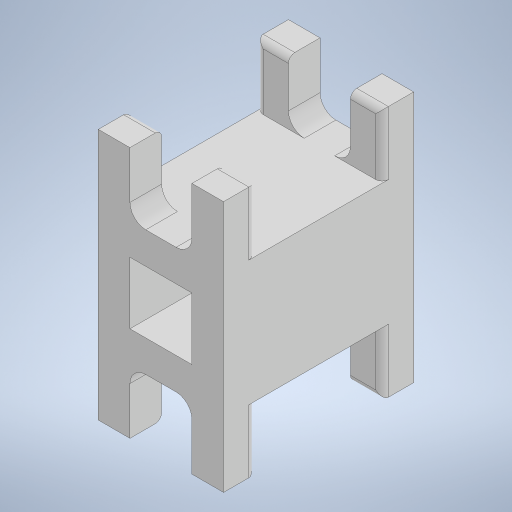
# Autodesk Inventor part: zigu3
Saved by Autodesk Inventor 2024.3 (Build 283343010, 343A)
## iProperties
Created: 2025-10-22
Part Number: zigu3
Material: 一般
Document SubType Name: Modeling
Designer: kshau
Density: 1 g/cm^3
Appearance: 既定
Author: kshau
Autodesk Inventor part; units mm, degrees
ref_plane "YZ Plane" through (0, 0, 0) normal (1, 0, 0) x (0, 1, 0)
ref_plane "XZ Plane" through (0, 0, 0) normal (0, 1, 0) x (-1, 0, 0)
ref_plane "XY Plane" through (0, 0, 0) normal (0, 0, 1) x (1, 0, 0)
sketch "スケッチ1" plane through (0, 0, 0) normal (0, 0, 1) x (1, 0, 0)
  line L0 (0, 0) -> (39.6, 0)
  line L1 (39.6, 0) -> (39.6, 39.6)
  line L2 (39.6, 39.6) -> (0, 39.6)
  line L3 (0, 39.6) -> (0, 0)
  line L4 (10, 29.6) -> (29.6, 29.6)
  line L5 (29.6, 29.6) -> (29.6, 10)
  line L6 (29.6, 10) -> (10, 10)
  line L7 (10, 10) -> (10, 29.6)
  dimension "d0" = 39.6
  dimension "d1" = 39.6
  dimension "d2" = 10
  dimension "d3" = 10
  dimension "d4" = 10
  dimension "d5" = 10
  constraints: 16 end point, 4 parallel, 2 horizontal, 2 perpendicular
  measures "d0" distance of L0.end L1.end
  measures "d1" distance of L1.end L2.end
  measures "d2" distance between parallel lines of L3 L7
  measures "d3" distance between parallel lines of L1 L5
  measures "d4" distance between parallel lines of L0 L6
  measures "d5" distance between parallel lines of L2 L4
extrude "押し出し1" add sketch "スケッチ1" along normal blind 20.05
sketch "スケッチ2" plane through (0, 0, 20.05) normal (0, 0, 1) x (1, 0, 0)
  line L0 (10, 10) -> (10, 29.6) projected
  line L1 (29.6, 29.6) -> (29.6, 10) projected
  line L2 (10, 10) -> (29.6, 10)
  line L3 (29.6, 10) -> (29.6, 29.6)
  line L4 (29.6, 29.6) -> (10, 29.6)
  line L5 (10, 29.6) -> (10, 10)
  line L6 (39.6, 39.6) -> (0, 39.6) projected
  line L7 (0, 39.6) -> (39.6, 39.6)
  line L8 (39.6, 39.6) -> (39.6, -20)
  line L9 (39.6, -20) -> (0, -20)
  line L10 (0, -20) -> (0, 39.6)
  line L11 (0, 0) -> (39.6, 0) projected
  line L12 (10, -20) -> (29.6, -20)
  line L13 (29.6, -20) -> (29.6, 0)
  line L14 (29.6, 0) -> (10, 0)
  line L15 (10, 0) -> (10, -20)
  line L16 (0, 0) -> (39.6, 0)
  line L17 (39.6, 0) -> (39.6, 59.6)
  line L18 (39.6, 59.6) -> (0, 59.6)
  line L19 (0, 59.6) -> (0, 0)
  line L20 (10, -20) -> (29.6, -20)
  line L21 (29.6, -20) -> (29.6, 59.6)
  line L22 (29.6, 59.6) -> (10, 59.6)
  line L23 (10, 59.6) -> (10, -20)
  point P0 (29.6, 10)
  point P1 (10, 0)
  point P2 (29.6, -20)
  point P3 (39.6, 39.6)
  point P4 (29.6, 39.6)
  point P5 (10, 39.6)
  point P6 (0, 39.6)
  dimension "d8" = 20
  dimension "d11" = 10
  dimension "d12" = 10
  dimension "d13" = 20
  constraints: 40 end point, 10 parallel, 6 point on line, 5 horizontal, 5 perpendicular
  measures "d8" distance between parallel lines of L11 L9
  measures "d11" distance between parallel lines of L10 L15
  measures "d12" distance between parallel lines of L8 L13
  measures "d13" distance between parallel lines of L6 L18
extrude "押し出し2" add sketch "スケッチ2" along normal blind 10 contours L23 L11 L10 L6 L0 | L2 L21 L11 L23 | L23 L6 L21 L4 | L1 L21 L6 L8 L11 | L15 L9 L10 L11 | L6 L19 L18 L23 | L11 L8 L9 L13 | L21 L18 L17 L6
mirror "ミラー1" about plane through (19.8, 19.8, 0) normal (0, 0, -1) of "押し出し1", "押し出し2"
fillet "フィレット1" radius 2 16 edges at (0, 49.6, -20.05) (5, 59.6, -20.05) (39.6, 49.6, -20.05) (34.6, 59.6, -20.05) (34.6, 59.6, 20.05) (39.6, 49.6, 20.05) (5, 59.6, 20.05) (0, 49.6, 20.05) (0, -10, 20.05) (5, -20, 20.05) (34.6, -20, 20.05) (39.6, -10, 20.05) (34.6, -20, -20.05) (39.6, -10, -20.05) (0, -10, -20.05) (5, -20, -20.05)
fillet "フィレット2" radius 5 8 edges at (10, 39.6, 25.05) (29.6, 39.6, 25.05) (10, 39.6, -25.05) (29.6, 39.6, -25.05) (10, 0, 25.05) (29.6, 0, 25.05) (29.6, 0, -25.05) (10, 0, -25.05)
